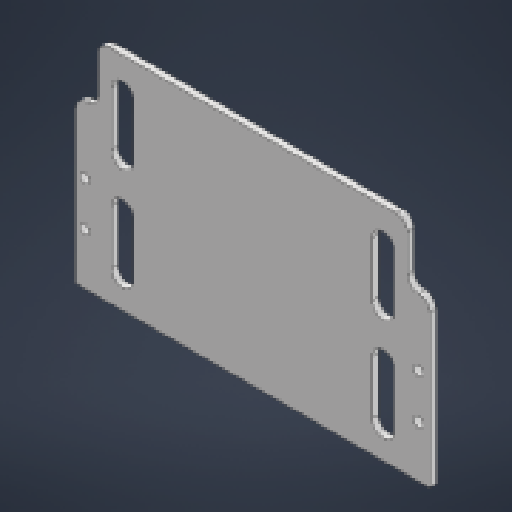
# Autodesk Inventor part: 前挡板2
Saved by Autodesk Inventor 2025 (Build 290162000, 162)
## iProperties
Created: 2024-12-28
Part Number: 前挡板2
Material: 常规
Document SubType Name: Modeling
Designer: HZD
Density: 1 g/cm^3
Appearance: 默认
Author: HZD
Autodesk Inventor part; units mm, degrees
ref_plane "YZ Plane" through (0, 0, 0) normal (1, 0, 0) x (0, 1, 0)
ref_plane "XZ Plane" through (0, 0, 0) normal (0, 1, 0) x (-1, 0, 0)
ref_plane "XY Plane" through (0, 0, 0) normal (0, 0, 1) x (1, 0, 0)
sketch "草图1" plane through (0, 0, 0) normal (0, 0, 1) x (1, 0, 0)
  line L0 (80, -50) -> (-80, -50)
  line L1 (-80, -50) -> (-80, 50)
  line L2 (-80, 50) -> (80, 50)
  line L3 (80, 50) -> (80, -50)
  line L4 (80, -50) -> (-80, 50) construction
  line L5 (-80, -50) -> (80, 50) construction
  point P0 (0, 0)
  dimension "d0" = 100
  dimension "d1" = 160
  constraints: 12 end point, 2 midpoint, 2 parallel, 1 horizontal, 1 perpendicular
  measures "d0" distance of L0.end L1.end
  measures "d1" distance of L1.end L2.end
extrude "拉伸1" add sketch "草图1" along normal blind 3
sketch "草图2" plane through (0, 0, 3) normal (0, 0, 1) x (1, 0, 0)
  line L0 (-70, 23.4843) -> (-70, 54.6776)
  line L1 (70, 15.0319) -> (70, 54.3435) projected
  line L2 (-80, 50) -> (-80, -50) projected
  line L3 (-80, 23.4843) -> (80.034, 23.4843)
  line L4 (80, 50) -> (-80, 50) projected
  line L5 (-80, 50) -> (-80, -50) projected
  line L6 (-80, -50) -> (80, -50) projected
  line L7 (80, -50) -> (80, 50) projected
  point P0 (0, 0)
  point P1 (80, 23.4843)
  point P2 (70, 50)
  point P3 (70, 23.4843)
  point P4 (-70, 50)
  dimension "d6" = 10
  dimension "d7" = 10
  constraints: 4 end point, 1 horizontal, 1 point on line
  measures "d6" distance between parallel lines of L2 L0
  measures "d7" distance between parallel lines of L7 L1
extrude "拉伸2" cut sketch "草图2" against normal blind 10 contours L3 L2 L4 L0 | L1 L4 L7 L3
fillet "圆角1" radius 5 6 edges at (-80, 23.4843, 1.5) (-70, 23.4843, 1.5) (-70, 50, 1.5) (70, 50, 1.5) (70, 23.4843, 1.5) (80, 23.4843, 1.5)
sketch "草图7" plane through (0, 0, 3) normal (0, 0, 1) x (1, 0, 0)
  circle A0 centre (75, -6.6525) radius 1.2 projected
  circle A1 centre (75, -26.6525) radius 1.2 projected
  circle A2 centre (-76, -6.6525) radius 1.2 projected
  circle A3 centre (-76, -26.6525) radius 1.2 projected
  circle A4 centre (-76, -6.6525) radius 2.2
  circle A5 centre (-76, -26.6525) radius 2.2
  circle A6 centre (75, -6.6525) radius 2.2
  circle A7 centre (75, -26.6525) radius 2.2
  point P0 (0, 0)
  dimension "d78" = 1
  dimension "d79" = 1
  dimension "d80" = 1
  dimension "d81" = 1
  constraints: 4 centre point
  measures "d78" radial gap between concentric circles of A2 A4
  measures "d79" radial gap between concentric circles of A3 A5
  measures "d80" radial gap between concentric circles of A0 A6
  measures "d81" radial gap between concentric circles of A1 A7
extrude "拉伸5" cut sketch "草图7" against normal blind 10 contours A0 | A1 | A2 | A3 | A4 | A5 | A6 | A7
sketch "草图6" plane through (0, 0, 3) normal (0, 0, 1) x (1, 0, 0)
  circle A0 centre (-0.337, 1.4402) radius 29.6824
  line L0 (58.9355, -11.5218) -> (58.9355, -35.9401) construction
  line L1 (53.9355, -11.5218) -> (53.9355, -35.9401)
  line L2 (63.9355, -35.9401) -> (63.9355, -11.5218)
  arc A1 (63.9355, -11.5218) -> (53.9355, -11.5218) centre (58.9355, -11.5218) ccw
  arc A2 (53.9355, -35.9401) -> (63.9355, -35.9401) centre (58.9355, -35.9401) ccw
  line L3 (58.9355, 34.7499) -> (58.9355, 10.3316) construction
  line L4 (53.9355, 34.7499) -> (53.9355, 10.3316)
  line L5 (63.9355, 10.3316) -> (63.9355, 34.7499)
  arc A3 (63.9355, 34.7499) -> (53.9355, 34.7499) centre (58.9355, 34.7499) ccw
  arc A4 (53.9355, 10.3316) -> (63.9355, 10.3316) centre (58.9355, 10.3316) ccw
  line L6 (65, 50) -> (-65, 50) projected
  line L7 (0, 50) -> (0, -49.5861)
  line L8 (-58.9355, -11.5218) -> (-58.9355, -35.9401) construction
  line L9 (-53.9355, -11.5218) -> (-53.9355, -35.9401)
  line L10 (-63.9355, -35.9401) -> (-63.9355, -11.5218)
  arc A5 (-53.9355, -11.5218) -> (-63.9355, -11.5218) centre (-58.9355, -11.5218) ccw
  arc A6 (-63.9355, -35.9401) -> (-53.9355, -35.9401) centre (-58.9355, -35.9401) ccw
  line L11 (-58.9355, 34.7499) -> (-58.9355, 10.3316) construction
  line L12 (-53.9355, 34.7499) -> (-53.9355, 10.3316)
  line L13 (-63.9355, 10.3316) -> (-63.9355, 34.7499)
  arc A7 (-53.9355, 34.7499) -> (-63.9355, 34.7499) centre (-58.9355, 34.7499) ccw
  arc A8 (-63.9355, 10.3316) -> (-53.9355, 10.3316) centre (-58.9355, 10.3316) ccw
  point P0 (0, 0)
  point P1 (58.9355, -23.7309)
  point P2 (58.9355, 22.5408)
  point P3 (-58.9355, -23.7309)
  point P4 (-58.9355, 22.5408)
  dimension "d70" = 5
  dimension "d71" = 5
  constraints: 34 end point, 16 point on circle, 14 symmetric about line, 9 centre point, 8 tangent, 3 midpoint, 3 vertical, 2 parallel, 1 coincident, 4 other
  measures "d70" radius of A1
  measures "d71" radius of A3
extrude "拉伸4" cut sketch "草图6" against normal blind 10 contours A1 L2 A2 L1 | A3 L5 A4 L4 | L9 A6 L10 A5 | L12 A8 L13 A7
sketch "草图5" plane through (0, 0, 3) normal (0, 0, 1) x (1, 0, 0)
  line L0 (-51.948, 44.2905) -> (50.6435, 44.2905) construction
  line L1 (50.6435, 44.2905) -> (50.6435, -58.301) construction
  line L2 (50.6435, -58.301) -> (-51.948, -58.301) construction
  line L3 (-51.948, -58.301) -> (-51.948, 44.2905) construction
  circle A0 centre (-0.337, 1.4402) radius 19.5793
  circle A1 centre (-0.337, 1.4402) radius 22.0126
  circle A2 centre (-0.1836, 17.5889) radius 1.0689
  circle A3 centre (14.0973, -7.3293) radius 1.2102
  circle A4 centre (-14.6768, -7.0871) radius 1.2453
  arc A5 (-1.5966, 22.3303) -> (-3.177, 23.2671) centre (-2.9305, 21.8816) ccw
  arc A6 (-1.5966, 22.3303) -> (1.2246, 22.333) centre (-0.1861, 22.4331) ccw
  arc A7 (2.2174, 23.304) -> (1.2246, 22.333) centre (2.87, 21.6437) ccw
  line L4 (-3.1076, 23.2777) -> (-2.7908, 20.865)
  line L5 (2.4336, 23.2777) -> (2.4336, 20.8224)
  arc A8 (-6.9604, 21.2925) -> (-8.7295, 21.7883) centre (-8.1327, 20.5138) ccw
  arc A9 (-6.9604, 21.2925) -> (-4.236, 22.0252) centre (-5.6246, 21.7569) ccw
  arc A10 (-3.5284, 23.2201) -> (-4.236, 22.0252) centre (-2.4683, 21.7854) ccw
  arc A11 (-11.8729, 18.9017) -> (-13.71, 18.9228) centre (-12.8037, 17.8462) ccw
  arc A12 (-11.8729, 18.9017) -> (-9.431, 20.3147) centre (-10.7028, 19.6961) ccw
  arc A13 (-9.0567, 21.652) -> (-9.431, 20.3147) centre (-7.6614, 20.5405) ccw
  arc A14 (-15.9992, 15.321) -> (-17.7792, 14.8659) centre (-16.6251, 14.0606) ccw
  arc A15 (-15.9992, 15.321) -> (-14.0062, 17.3179) centre (-15.0746, 16.3912) ccw
  arc A16 (-13.9908, 18.7065) -> (-14.0062, 17.3179) centre (-12.3554, 17.994) ccw
  arc A17 (-19.0582, 10.7944) -> (-20.6597, 9.8941) centre (-19.3365, 9.4149) ccw
  arc A18 (-19.0582, 10.7944) -> (-17.6499, 13.239) centre (-18.442, 12.0674) ccw
  arc A19 (-17.9944, 14.5843) -> (-17.6499, 13.239) centre (-16.2303, 14.3193) ccw
  arc A20 (-20.8413, 5.6302) -> (-22.1553, 4.3462) centre (-20.7531, 4.2257) ccw
  arc A21 (-20.8413, 5.6302) -> (-20.1137, 8.356) centre (-20.5756, 7.0193) ccw
  arc A22 (-20.7947, 9.5663) -> (-20.1137, 8.356) centre (-19.0221, 9.767) ccw
  arc A23 (-21.2271, 0.1806) -> (-22.164, -1.3998) centre (-20.7784, -1.1533) ccw
  arc A24 (-21.2271, 0.1806) -> (-21.2298, 3.0018) centre (-21.33, 1.5911) ccw
  arc A25 (-22.2009, 3.9946) -> (-21.2298, 3.0018) centre (-20.5406, 4.6472) ccw
  arc A26 (-20.1893, -5.1833) -> (-20.6852, -6.9523) centre (-19.4107, -6.3555) ccw
  arc A27 (-20.1893, -5.1833) -> (-20.9221, -2.4589) centre (-20.6537, -3.8474) ccw
  arc A28 (-22.117, -1.7512) -> (-20.9221, -2.4589) centre (-20.6822, -0.6911) ccw
  arc A29 (-17.7986, -10.0958) -> (-17.8197, -11.9328) centre (-16.7431, -11.0265) ccw
  arc A30 (-17.7986, -10.0958) -> (-19.2115, -7.6538) centre (-18.5929, -8.9256) ccw
  arc A31 (-20.5489, -7.2796) -> (-19.2115, -7.6538) centre (-19.4374, -5.8843) ccw
  arc A32 (-14.2179, -14.2221) -> (-13.7628, -16.002) centre (-12.9574, -14.8479) ccw
  arc A33 (-14.2179, -14.2221) -> (-16.2147, -12.229) centre (-15.288, -13.2974) ccw
  arc A34 (-17.6033, -12.2137) -> (-16.2147, -12.229) centre (-16.8908, -10.5782) ccw
  arc A35 (-9.6912, -17.281) -> (-8.791, -18.8825) centre (-8.3117, -17.5594) ccw
  arc A36 (-9.6912, -17.281) -> (-12.1358, -15.8727) centre (-10.9642, -16.6648) ccw
  arc A37 (-13.4811, -16.2173) -> (-12.1358, -15.8727) centre (-13.2162, -14.4531) ccw
  arc A38 (-4.5271, -19.0642) -> (-3.243, -20.3781) centre (-3.1226, -18.976) ccw
  arc A39 (-4.5271, -19.0642) -> (-7.2529, -18.3366) centre (-5.9162, -18.7985) ccw
  arc A40 (-8.4632, -19.0176) -> (-7.2529, -18.3366) centre (-8.6639, -17.245) ccw
  arc A41 (0.9226, -19.45) -> (2.503, -20.3868) centre (2.2564, -19.0013) ccw
  arc A42 (0.9226, -19.45) -> (-1.8987, -19.4527) centre (-0.4879, -19.5528) ccw
  arc A43 (-2.8914, -20.4237) -> (-1.8987, -19.4527) centre (-3.5441, -18.7634) ccw
  arc A44 (6.2864, -18.4122) -> (8.0554, -18.908) centre (7.4587, -17.6335) ccw
  arc A45 (6.2864, -18.4122) -> (3.562, -19.1449) centre (4.9506, -18.8766) ccw
  arc A46 (2.8544, -20.3398) -> (3.562, -19.1449) centre (1.7943, -18.9051) ccw
  arc A47 (11.1989, -16.0214) -> (13.036, -16.0425) centre (12.1297, -14.9659) ccw
  arc A48 (11.1989, -16.0214) -> (8.757, -17.4344) centre (10.0288, -16.8158) ccw
  arc A49 (8.3827, -18.7717) -> (8.757, -17.4344) centre (6.9874, -17.6602) ccw
  arc A50 (15.3252, -12.4407) -> (17.1051, -11.9856) centre (15.9511, -11.1803) ccw
  arc A51 (15.3252, -12.4407) -> (13.3322, -14.4376) centre (14.4005, -13.5109) ccw
  arc A52 (13.3168, -15.8262) -> (13.3322, -14.4376) centre (11.6814, -15.1137) ccw
  arc A53 (18.3842, -7.9141) -> (19.9857, -7.0138) centre (18.6625, -6.5346) ccw
  arc A54 (18.3842, -7.9141) -> (16.9759, -10.3587) centre (17.768, -9.1871) ccw
  arc A55 (17.3204, -11.704) -> (16.9759, -10.3587) centre (15.5563, -11.439) ccw
  arc A56 (20.1673, -2.7499) -> (21.4812, -1.4659) centre (20.0791, -1.3454) ccw
  arc A57 (20.1673, -2.7499) -> (19.4397, -5.4757) centre (19.9016, -4.139) ccw
  arc A58 (20.1207, -6.686) -> (19.4397, -5.4757) centre (18.3481, -6.8867) ccw
  arc A59 (20.5531, 2.6997) -> (21.4899, 4.2801) centre (20.1044, 4.0336) ccw
  arc A60 (20.5531, 2.6997) -> (20.5558, -0.1215) centre (20.656, 1.2892) ccw
  arc A61 (21.5268, -1.1143) -> (20.5558, -0.1215) centre (19.8666, -1.7669) ccw
  arc A62 (19.5153, 8.0636) -> (20.0111, 9.8326) centre (18.7366, 9.2358) ccw
  arc A63 (19.5153, 8.0636) -> (20.2481, 5.3392) centre (19.9797, 6.7277) ccw
  arc A64 (21.443, 4.6315) -> (20.2481, 5.3392) centre (20.0082, 3.5714) ccw
  arc A65 (17.1246, 12.9761) -> (17.1457, 14.8131) centre (16.0691, 13.9068) ccw
  arc A66 (17.1246, 12.9761) -> (18.5375, 10.5341) centre (17.9189, 11.8059) ccw
  arc A67 (19.8749, 10.1599) -> (18.5375, 10.5341) centre (18.7633, 8.7646) ccw
  arc A68 (13.5439, 17.1024) -> (13.0888, 18.8823) centre (12.2834, 17.7283) ccw
  arc A69 (13.5439, 17.1024) -> (15.5407, 15.1093) centre (14.614, 16.1777) ccw
  arc A70 (16.9293, 15.094) -> (15.5407, 15.1093) centre (16.2168, 13.4585) ccw
  arc A71 (9.0172, 20.1613) -> (8.1169, 21.7628) centre (7.6377, 20.4397) ccw
  arc A72 (9.0172, 20.1613) -> (11.4618, 18.753) centre (10.2902, 19.5451) ccw
  arc A73 (12.8071, 19.0976) -> (11.4618, 18.753) centre (12.5422, 17.3335) ccw
  arc A74 (3.8531, 21.9445) -> (2.569, 23.2584) centre (2.4485, 21.8563) ccw
  arc A75 (3.8531, 21.9445) -> (6.5789, 21.2169) centre (5.2422, 21.6788) ccw
  arc A76 (7.7892, 21.8979) -> (6.5789, 21.2169) centre (7.9898, 20.1253) ccw
  circle A77 centre (-0.337, 1.4402) radius 17.3264
  arc A78 (-1.8119, 16.3912) -> (1.4108, 16.5709) centre (-0.2439, 17.2588) ccw
  line L6 (-1.8119, 16.3912) -> (-3.3302, 18.506)
  line L7 (1.4108, 16.5709) -> (2.5167, 18.5299)
  line L8 (-16.4097, -5.0307) -> (-13.9908, -5.0307)
  line L9 (-13.4922, -9.8356) -> (-12.6482, -7.9141)
  arc A79 (-12.6482, -7.9141) -> (-13.9908, -5.0307) centre (-14.3731, -6.963) ccw
  line L10 (12.9811, -9.6427) -> (11.9394, -7.9141)
  arc A80 (13.1454, -5.3295) -> (11.9394, -7.9141) centre (13.7218, -7.1721) ccw
  line L11 (13.1454, -5.3295) -> (15.7357, -5.0307)
  line L12 (-9.9945, 15.2423) -> (9.7915, 15.2423)
  line L13 (9.7915, 15.2423) -> (9.7915, 12.3918)
  line L14 (9.7915, 12.3918) -> (4.8774, 12.3918)
  line L15 (4.8774, 12.3918) -> (4.8774, 11.3614)
  line L16 (4.8774, 11.3614) -> (-0.1015, 3.7166)
  line L17 (-0.1015, 3.7166) -> (4.8774, 5.6302)
  line L18 (4.8774, 5.6302) -> (4.8774, -10.799)
  line L19 (4.8774, -10.799) -> (9.9178, -10.799)
  line L20 (-10.2582, -10.5782) -> (-10.3245, -13.73)
  line L21 (-10.3245, -13.73) -> (8.2621, -13.73)
  line L22 (-10.2582, -10.5782) -> (-4.859, -10.5782)
  line L23 (-4.859, -10.5782) -> (-4.859, -9.8356)
  line L24 (-4.859, -9.8356) -> (0.725, -0.9592)
  line L25 (0.725, -0.9592) -> (-4.859, -4.139)
  line L26 (-4.859, -4.139) -> (-4.9409, 11.6269)
  line L27 (-4.9409, 11.6269) -> (-9.9945, 11.6007)
  line L28 (-9.9945, 11.6007) -> (-9.9945, 15.2423)
  line L29 (-6.5155, -6.1315) -> (-3.3302, -4.6028)
  line L30 (-3.3302, -4.6028) -> (-6.4171, -9.3424)
  line L31 (-6.4171, -9.3424) -> (-6.5155, -6.1315)
  line L32 (2.7649, 6.2064) -> (5.9307, 7.7259)
  line L33 (5.9307, 7.7259) -> (5.9307, 10.7944)
  line L34 (5.9307, 10.7944) -> (2.7649, 6.2064)
  line L35 (9.9178, -10.799) -> (9.9178, -13.73)
  point P0 (-8.6651, 21.8165)
  point P1 (-13.6551, 18.9667)
  point P2 (-17.7376, 14.9225)
  point P3 (-20.6341, 9.9595)
  point P4 (-22.1475, 4.416)
  point P5 (-22.1745, -1.3304)
  point P6 (-20.7134, -6.888)
  point P7 (-17.8636, -11.878)
  point P8 (-13.8194, -15.9604)
  point P9 (-8.8564, -18.857)
  point P10 (-3.3128, -20.3703)
  point P11 (2.4336, -20.3974)
  point P12 (7.9911, -18.9362)
  point P13 (12.9811, -16.0864)
  point P14 (17.0635, -12.0422)
  point P15 (19.9601, -7.0792)
  point P16 (21.4735, -1.5357)
  point P17 (21.5005, 4.2107)
  point P18 (20.0393, 9.7683)
  point P19 (17.1895, 14.7583)
  point P20 (13.1454, 18.8407)
  point P21 (8.1824, 21.7373)
  point P22 (2.6388, 23.2506)
  point P23 (-3.5284, 23.2201)
  point P24 (-8.6651, 21.8165)
  point P25 (-13.6551, 18.9667)
  point P26 (-13.9908, 18.7065)
  point P27 (-17.7376, 14.9225)
  point P28 (-17.9944, 14.5843)
  point P29 (-20.6341, 9.9595)
  point P30 (-22.1475, 4.416)
  point P31 (-22.1745, -1.3304)
  point P32 (-22.117, -1.7512)
  point P33 (-20.7134, -6.888)
  point P34 (-17.8636, -11.878)
  point P35 (-17.6033, -12.2137)
  point P36 (-13.8194, -15.9604)
  point P37 (-8.8564, -18.857)
  point P38 (-3.3128, -20.3703)
  point P39 (-2.8914, -20.4237)
  point P40 (2.4336, -20.3974)
  point P41 (2.8544, -20.3398)
  point P42 (7.9911, -18.9362)
  point P43 (8.3827, -18.7717)
  point P44 (12.9811, -16.0864)
  point P45 (17.0635, -12.0422)
  point P46 (19.9601, -7.0792)
  point P47 (20.1207, -6.686)
  point P48 (21.4735, -1.5357)
  point P49 (21.5005, 4.2107)
  point P50 (21.443, 4.6315)
  point P51 (20.0393, 9.7683)
  point P52 (19.8749, 10.1599)
  point P53 (17.1895, 14.7583)
  point P54 (16.9293, 15.094)
  point P55 (13.1454, 18.8407)
  point P56 (8.1824, 21.7373)
  point P57 (7.7892, 21.8979)
  point P58 (2.6388, 23.2506)
  point P59 (-10.3035, -12.7328)
  point P60 (-8.7078, -13.73)
  point P61 (8.0337, -13.73)
  point P62 (9.9178, -12.5256)
  dimension "d45" = 39.1585
  dimension "d51" = 360
  constraints: 182 point on circle, 80 centre point, 64 end point, 6 perpendicular, 4 horizontal, 3 point on line, 2 coincident, 2 parallel, 2 vertical, 1 tangent, 273 other
  measures "d45" diameter of A0
